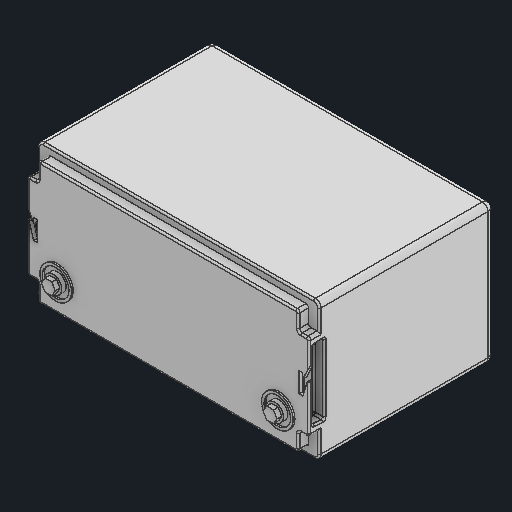
# Autodesk Inventor part: XznyCompactSeriesX
Saved by Autodesk Inventor 2025.2 (Build 292293000, 293)
## iProperties
Created: 2025-11-05
Part Number: XznyCompactSeriesX
Material: Generic
Document SubType Name: Modeling
Designer: valer
Density: 1 g/cm^3
Appearance: Default
Author: valer
Autodesk Inventor part; units mm, degrees
ref_plane "YZ Plane" through (0, 0, 0) normal (1, 0, 0) x (0, 1, 0)
ref_plane "XZ Plane" through (0, 0, 0) normal (0, 1, 0) x (-1, 0, 0)
ref_plane "XY Plane" through (0, 0, 0) normal (0, 0, 1) x (1, 0, 0)
sketch "Base" plane through (0, 0, 0) normal (0, 0, 1) x (1, 0, 0)
  line L0 (164, -80.25) -> (-164, -80.25)
  line L1 (-164, -80.25) -> (-164, 80.25)
  line L2 (-164, 80.25) -> (164, 80.25)
  line L3 (164, 80.25) -> (164, -80.25)
  line L4 (164, -80.25) -> (-164, 80.25) construction
  line L5 (-164, -80.25) -> (164, 80.25) construction
  point P0 (0, 0)
  dimension "d0" = 328
  dimension "d1" = 160.5
  constraints: 12 end point, 2 midpoint, 2 parallel, 1 horizontal, 1 perpendicular
  measures "d0" distance of L1.end L2.end
  measures "d1" distance of L2.end L0.start
extrude "BaseFeature" add sketch "Base" along normal blind 203
fillet "BaseFilletsFeature" radius 6.5 8 edges at (-164, -80.25, 101.5) (164, -80.25, 101.5) (164, 80.25, 101.5) (-164, 80.25, 101.5) (0, -80.25, 0) (164, 0, 0) (-164, 0, 0) (0, 80.25, 0)
sketch "Lid" plane through (0, 0, 203) normal (0, 0, 1) x (1, 0, 0)
  arc A0 (-164, -73.75) -> (-157.5, -80.25) centre (-157.5, -73.75) ccw projected
  line L0 (-157.5, -80.25) -> (157.5, -80.25) projected
  arc A1 (157.5, -80.25) -> (164, -73.75) centre (157.5, -73.75) ccw projected
  line L1 (164, -73.75) -> (164, 73.75) projected
  arc A2 (164, 73.75) -> (157.5, 80.25) centre (157.5, 73.75) ccw projected
  line L2 (157.5, 80.25) -> (-157.5, 80.25) projected
  arc A3 (-157.5, 80.25) -> (-164, 73.75) centre (-157.5, 73.75) ccw projected
  line L3 (-164, 73.75) -> (-164, -73.75) projected
  line L4 (-164, 71.5) -> (164, 71.5)
  line L5 (164, 71.5) -> (164, -71.5)
  line L6 (164, -71.5) -> (-164, -71.5)
  line L7 (-164, -71.5) -> (-164, 71.5)
  line L8 (-231.4847, 0) -> (231.4847, 0) construction
  line L9 (-164, 50) -> (-151.5, 50)
  line L10 (-151.5, 50) -> (-151.5, 71.5)
  line L11 (-164, -50) -> (-151.5, -50)
  line L12 (-151.5, -50) -> (-151.5, -71.5)
  line L13 (0, -114.2347) -> (0, 114.2347) construction
  line L14 (164, 50) -> (151.5, 50)
  line L15 (151.5, 50) -> (151.5, 71.5)
  line L16 (164, -50) -> (151.5, -50)
  line L17 (151.5, -50) -> (151.5, -71.5)
  point P0 (0, 0)
  point P1 (-164, 0)
  point P2 (151.5, -71.5)
  point P3 (164, -50)
  point P4 (151.5, 71.5)
  point P5 (-164, 50)
  dimension "d5" = 8.75
  dimension "d6" = 143
  dimension "d7" = 100
  dimension "d8" = 12.5
  constraints: 24 end point, 9 symmetric about line, 3 perpendicular, 3 point on line, 2 collinear, 2 parallel, 1 horizontal, 1 midpoint
  measures "d5" distance between parallel lines of L2 L4
  measures "d6" distance between parallel lines of L6 L4
  measures "d7" distance between parallel lines of L11 L9
  measures "d8" distance of L9.start L9.end
extrude "LidFeature" add sketch "Lid" along normal blind 12 contours L3 L9 L10 L4 L15 L14 L1 L16 L17 L6 L12 L11
fillet "LidFilletsFeature" radius 3 12 edges at (-151.5, -71.5, 209) (-151.5, 71.5, 209) (-151.5, -50, 209) (-164, -50, 209) (-151.5, 50, 209) (-164, 50, 209) (151.5, 71.5, 209) (151.5, 50, 209) (164, 50, 209) (164, -50, 209) (151.5, -71.5, 209) (151.5, -50, 209)
fillet "TopFilletsFeature" radius 2 38 edges at (162.0962, -78.3462, 203) (0, -80.25, 203) (-162.0962, -78.3462, 203) (-164, -48.5, 203) (-164, -61.875, 203) (164, -61.875, 203) (164, -48.5, 203) (162.0962, 78.3462, 203) (0, 80.25, 203) (-162.0962, 78.3462, 203) (-164, 48.5, 203) (-164, 61.875, 203) (164, 48.5, 203) (164, 61.875, 203) (150.6213, -70.6213, 215) (151.5, -60.75, 215) (152.3787, -50.8787, 215) (157.75, -50, 215) (163.1213, -49.1213, 215) (164, 0, 215) (163.1213, 49.1213, 215) (157.75, 50, 215) (152.3787, 50.8787, 215) (151.5, 60.75, 215) (150.6213, 70.6213, 215) (0, 71.5, 215) (-150.6213, 70.6213, 215) (-151.5, 60.75, 215) (-152.3787, 50.8787, 215) (-157.75, 50, 215) (-163.1213, 49.1213, 215) (-164, 0, 215) (-163.1213, -49.1213, 215) (-157.75, -50, 215) (-152.3787, -50.8787, 215) (-151.5, -60.75, 215) (-150.6213, -70.6213, 215) (0, -71.5, 215)
sketch "ContactRidges" plane through (0, 0, 215) normal (0, 0, 1) x (1, 0, 0)
  circle A0 centre (-129.1, -39.4) radius 18.4
  line L0 (-229.6, 0) -> (229.6, 0) construction
  line L1 (0, -112.35) -> (0, 112.35) construction
  circle A1 centre (129.1, -39.4) radius 18.4
  line L2 (-147.5, -57.8) -> (-110.7, -57.8) construction
  line L3 (-110.7, -57.8) -> (-110.7, -21) construction
  line L4 (-110.7, -21) -> (-147.5, -21) construction
  line L5 (-147.5, -21) -> (-147.5, -57.8) construction
  line L6 (-147.5, -57.8) -> (-110.7, -21) construction
  line L7 (-110.7, -57.8) -> (-147.5, -21) construction
  line L8 (-164, 47) -> (-164, -47) projected
  line L9 (148.5, 71.5) -> (-148.5, 71.5) projected
  point P0 (0, 0)
  dimension "d13" = 36.8
  dimension "d14" = 16.5
  dimension "d15" = 92.5
  constraints: 12 end point, 2 centre point, 2 midpoint, 2 parallel, 2 tangent, 1 horizontal, 1 perpendicular, 1 symmetric about line, 1 other
  measures "d13" diameter of A0
  measures "d14" distance between parallel lines of L8 L5
  measures "d15" distance between parallel lines of L9 L4
extrude "ContactRidgesFeature" add sketch "ContactRidges" along normal blind 2
sketch "RidgeInside" plane through (-129.1, -39.4, 217) normal (0, 0, 1) x (1, 0, 0)
  circle A0 centre (0, 0) radius 18.4 projected
  circle A1 centre (258.2, 0) radius 18.4 projected
  circle A2 centre (0, 0) radius 15.4
  circle A3 centre (258.2, 0) radius 15.4
  point P0 (129.1, 39.4)
  dimension "d18" = 3
  dimension "d19" = 3
  constraints: 2 centre point, 2 coincident
  measures "d18" radial gap between concentric circles of A0 A2
  measures "d19" radial gap between concentric circles of A1 A3
extrude "RidgeInsideFeature" cut sketch "RidgeInside" against normal up to surface (2 mm away) contours A2 | A3
sketch "Contacts" plane through (-129.1, -39.4, 215) normal (0, 0, 1) x (1, 0, 0)
  circle A0 centre (0, 0) radius 15.4 projected
  circle A1 centre (258.2, 0) radius 15.4 projected
  circle A2 centre (0, 0) radius 10.125
  circle A3 centre (258.2, 0) radius 10.125
  point P0 (129.1, 39.4)
  dimension "d22" = 20.25
  constraints: 2 centre point, 2 coincident, 1 equal radius
  measures "d22" diameter of A2
extrude "ContactsFeature" add sketch "Contacts" along normal blind 5 contours A2 | A3
sketch "Bolts" plane through (-129.1, -39.4, 220) normal (0, 0, 1) x (1, 0, 0)
  circle A0 centre (0, 0) radius 10.125 projected
  circle A1 centre (258.2, 0) radius 10.125 projected
  line L0 (4.0415, 7) -> (8.0829, 0)
  line L1 (8.0829, 0) -> (4.0415, -7)
  line L2 (4.0415, -7) -> (-4.0415, -7)
  line L3 (-4.0415, -7) -> (-8.0829, 0)
  line L4 (-8.0829, 0) -> (-4.0415, 7)
  line L5 (-4.0415, 7) -> (4.0415, 7)
  line L6 (-100.5026, 39.4) -> (358.7026, 39.4) construction
  line L7 (262.2415, 7) -> (266.2829, 0)
  line L8 (266.2829, 0) -> (262.2415, -7)
  line L9 (262.2415, -7) -> (254.1585, -7)
  line L10 (254.1585, -7) -> (250.1171, 0)
  line L11 (250.1171, 0) -> (254.1585, 7)
  line L12 (254.1585, 7) -> (262.2415, 7)
  point P0 (129.1, 39.4)
  dimension "d25" = 14
  constraints: 24 end point, 2 coincident, 2 parallel, 1 collinear, 26 other
  measures "d25" distance between parallel lines of L2 L5
extrude "BoltsFeature" add sketch "Bolts" along normal blind 5.5 contours L0 L1 L2 L3 L4 L5 | L7 L8 L9 L10 L11 L12
sketch "MountSlits" plane through (0, 0, 215) normal (0, 0, 1) x (1, 0, 0)
  line L0 (-229.6, 0) -> (229.6, 0) construction
  line L1 (-156.75, -11.75) -> (-152.25, -11.75)
  line L2 (-152.25, -11.75) -> (-152.25, 11.75)
  line L3 (-152.25, 11.75) -> (-156.75, 11.75)
  line L4 (-156.75, 11.75) -> (-156.75, -11.75)
  line L5 (-156.75, -11.75) -> (-152.25, 11.75) construction
  line L6 (-152.25, -11.75) -> (-156.75, 11.75) construction
  line L7 (-161, -50) -> (-154.5, -50) projected
  line L8 (-164, 47) -> (-164, -47) projected
  line L9 (-156.75, -11.75) -> (-162, 5.25)
  line L10 (-162, -47) -> (-162, 47) projected
  line L11 (-156.75, 5.25) -> (-156.75, 5.25)
  line L12 (-162, 5.25) -> (-164, 5.25)
  line L13 (-162, 5.25) -> (-156.75, 5.25) construction
  line L14 (-154.5, 50) -> (-161, 50) projected
  line L15 (-156.75, 5.25) -> (-164, 20.75)
  line L16 (-156.75, 5.25) -> (-156.75, -11.75) construction
  line L17 (0, -112.35) -> (0, 112.35) construction
  line L18 (156.75, -11.75) -> (152.25, -11.75)
  line L19 (152.25, -11.75) -> (152.25, 11.75)
  line L20 (152.25, 11.75) -> (156.75, 11.75)
  line L21 (156.75, 11.75) -> (156.75, -11.75)
  line L22 (156.75, -11.75) -> (162, 5.25)
  line L23 (162, 5.25) -> (164, 5.25)
  line L24 (156.75, 5.25) -> (164, 20.75)
  line L25 (164, -47) -> (164, 47) projected
  point P0 (0, 0)
  point P1 (-154.5, 0)
  point P2 (-156.75, 5.25)
  dimension "d29" = 4.5
  dimension "d34" = 23.5
  dimension "d39" = 15.5
  dimension "d41" = 7.25
  dimension "d42" = 17
  constraints: 38 end point, 8 symmetric about line, 5 point on line, 3 perpendicular, 2 horizontal, 2 midpoint, 1 parallel, 1 vertical
  measures "d29" distance between parallel lines of L2 L4
  measures "d34" distance of L1.end L2.end
  measures "d39" distance of L15.end L12.end
  measures "d41" distance between parallel lines of L8 L4
  measures "d42" distance between parallel lines of L1 L12
extrude "MountSlitsFeature" cut sketch "MountSlits" against normal up to surface (12 mm away)
sketch "MountIndents" plane through (-164, -73.75, 6.5) normal (-1, 0, 0) x (0, 0, 1)
  line L0 (204, 113.75) -> (204, 33.75)
  line L1 (204, 33.75) -> (190.5, 32.75)
  line L2 (190.5, 32.75) -> (190.5, 114.75)
  line L3 (190.5, 114.75) -> (204, 113.75)
  line L4 (208.5, 90.2241) -> (208.5, 120.75) projected
  line L5 (-51.7, 73.75) -> (264.7, 73.75) construction
  point P0 (-6.5, 73.75)
  point P1 (204, 73.75)
  point P2 (190.5, 73.75)
  dimension "d47" = 4.5
  dimension "d48" = 13.5
  dimension "d49" = 80
  dimension "d50" = 82
  constraints: 8 end point, 2 midpoint, 2 point on line, 1 parallel, 1 vertical
  measures "d47" distance between parallel lines of L4 L0
  measures "d48" distance between parallel lines of L2 L0
  measures "d49" distance of L0.start L0.end
  measures "d50" distance of L1.end L2.end
extrude "MountIndentFeature" cut sketch "MountIndents" against normal up to surface (12.5 mm away)
mirror "MountIndentsMirrorFeature" about plane through (0, 0, 0) normal (1, 0, 0) of "MountIndentFeature"
fillet "MountIndentFilletsFeature" radius 2 13 edges at (-164, 40.5, 203.75) (-164, 0, 197) (-164, -40.5, 203.75) (-164, -17.375, 210.5) (-164, 30.375, 210.5) (-151.5, 0, 210.5) (-151.5, -40.5, 203.75) (-151.5, 40.5, 203.75) (-151.5, 0, 197) (-157.75, 41, 197) (-157.75, -41, 197) (-157.75, -40, 210.5) (-157.75, 40, 210.5)
fillet "MountIndentFillets2Feature" radius 2 8 edges at (151.5, -40.5, 203.75) (151.5, 0, 197) (151.5, 40.5, 203.75) (151.5, 0, 210.5) (157.75, 40, 210.5) (157.75, -40, 210.5) (157.75, -41, 197) (157.75, 41, 197)
fillet "RestFilletsFeature" radius 2 9 edges at (164, -40.3119, 197.639) (164, -40.4891, 203.8977) (164, -39.5036, 209.9655) (164, -16.4463, 210.5) (164, 40.3119, 197.639) (164, 40.4891, 203.8977) (164, 39.5036, 209.9655) (164, 29.4463, 210.5) (164, 0, 197)
body "Solid1"
